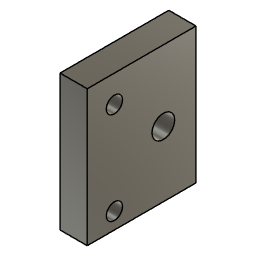
Car Chasis v11 (Autodesk Fusion 360 archive; units mm, degrees)
design "Motor Mount"
Autodesk Fusion 360 part; units mm, degrees
sketch "Sketch1" plane through (0, 0, 0) normal (0, 0, 1) x (1, 0, 0)
  line L0 (0, -50) -> (-40, -50)
  line L1 (-40, -50) -> (-40, 0)
  line L2 (-40, 0) -> (0, 0)
  line L3 (0, 0) -> (0, -50)
  constraint horizontal L0
  constraint vertical L1
  constraint horizontal L2
  constraint vertical L3
extrude "Extrude1" add sketch "Sketch1" along normal blind 8
sketch "Sketch2" plane through (0, 0, 8) normal (0, 0, 1) x (-1, 0, 0)
  line L0 (0, 0) -> (40, 0)
  line L1 (40, 0) -> (40, 50)
  line L2 (40, 50) -> (0, 50)
  line L3 (0, 50) -> (0, 0)
  line L4 (21, 0) -> (16, 0)
  line L5 (16, 0) -> (16, 20)
  line L6 (16, 20) -> (21, 20)
  line L7 (21, 20) -> (21, 0)
  dimension "d3" = 5
  dimension "d4" = 20
  constraint horizontal L4
  constraint vertical L5
  constraint horizontal L6
  constraint vertical L7
  constraint coincident L0 L4.start
  measures "d3" distance of L4.start L4.end
  measures "d4" distance of L4.start L6.end
extrude "Extrude2" add sketch "Sketch2" along normal blind 25 contours L0 L4 L5 L6 L7
hole "Hole1" at (-16, -15, 11) direction (-1, 0, 0) diameter 3 depth 6 tip angle 118
hole "Hole2" at (-16, -15, 28) direction (-1, 0, 0) diameter 3 depth 6 tip angle 118
hole "Hole3" at (-16, -6, 20) direction (-1, 0, 0) diameter 4.2 depth 6 tip angle 118
extrude "Extrude3" cut 1 faces at (-13.3333, -33.3333, 0) along direction (0, 0, 1) blind 8
